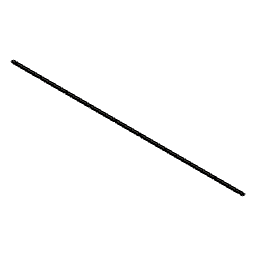
Stringers (Autodesk Fusion 360 design; units mm, degrees)
Autodesk Fusion 360 part; units mm, degrees
sketch "Sketch1" plane through (0, 0, 0) normal (0, 0, 1) x (1, 0, 0)
  line L0 (15.9527, 9.277) -> (765.9527, 9.277)
  line L1 (765.9527, 9.277) -> (765.9527, 3.277)
  line L2 (15.9527, 3.277) -> (15.9527, 9.277)
  line L3 (28.9527, 3.277) -> (28.9527, 6.277)
  line L4 (28.9527, 6.277) -> (25.9527, 6.277)
  line L5 (25.9527, 6.277) -> (25.9527, 3.277)
  line L6 (25.9527, 3.277) -> (15.9527, 3.277)
  line L7 (109.7327, 3.277) -> (109.7327, 6.277)
  line L8 (109.7327, 6.277) -> (106.7327, 6.277)
  line L9 (106.7327, 6.277) -> (106.7327, 3.277)
  line L10 (106.7327, 3.277) -> (28.9527, 3.277)
  line L11 (190.5127, 3.277) -> (190.5127, 6.277)
  line L12 (190.5127, 6.277) -> (187.5127, 6.277)
  line L13 (187.5127, 6.277) -> (187.5127, 3.277)
  line L14 (187.5127, 3.277) -> (109.7327, 3.277)
  line L15 (271.2927, 3.277) -> (271.2927, 6.277)
  line L16 (271.2927, 6.277) -> (268.2927, 6.277)
  line L17 (268.2927, 6.277) -> (268.2927, 3.277)
  line L18 (268.2927, 3.277) -> (190.5127, 3.277)
  line L19 (352.0727, 3.277) -> (352.0727, 6.277)
  line L20 (352.0727, 6.277) -> (349.0727, 6.277)
  line L21 (349.0727, 6.277) -> (349.0727, 3.277)
  line L22 (349.0727, 3.277) -> (271.2927, 3.277)
  line L23 (432.8527, 3.277) -> (432.8527, 6.277)
  line L24 (432.8527, 6.277) -> (429.8527, 6.277)
  line L25 (429.8527, 6.277) -> (429.8527, 3.277)
  line L26 (429.8527, 3.277) -> (352.0727, 3.277)
  line L27 (513.6327, 3.277) -> (513.6327, 6.277)
  line L28 (513.6327, 6.277) -> (510.6327, 6.277)
  line L29 (510.6327, 6.277) -> (510.6327, 3.277)
  line L30 (510.6327, 3.277) -> (432.8527, 3.277)
  line L31 (594.4127, 3.277) -> (594.4127, 6.277)
  line L32 (594.4127, 6.277) -> (591.4127, 6.277)
  line L33 (591.4127, 6.277) -> (591.4127, 3.277)
  line L34 (591.4127, 3.277) -> (513.6327, 3.277)
  line L35 (675.1927, 3.277) -> (675.1927, 6.277)
  line L36 (675.1927, 6.277) -> (672.1927, 6.277)
  line L37 (672.1927, 6.277) -> (672.1927, 3.277)
  line L38 (672.1927, 3.277) -> (594.4127, 3.277)
  line L39 (675.1927, 3.277) -> (752.9727, 3.277)
  line L40 (755.9727, 3.277) -> (755.9727, 6.277)
  line L41 (755.9727, 6.277) -> (752.9727, 6.277)
  line L42 (752.9727, 6.277) -> (752.9727, 3.277)
  line L43 (765.9527, 3.277) -> (755.9727, 3.277)
  line L44 (752.9727, 3.277) -> (675.1927, 3.277)
  dimension "d1" = 750
  dimension "d2" = 6
  constraint horizontal L0
  constraint vertical L1
  constraint horizontal L43
  constraint vertical L2
  constraint vertical L3
  constraint horizontal L4
  constraint vertical L5
  constraint collinear L6 L43
  constraint equal L4 L5
  constraint vertical L7
  constraint horizontal L8
  constraint vertical L9
  constraint collinear L10 L43
  constraint equal L7 L8
  constraint vertical L11
  constraint horizontal L12
  constraint vertical L13
  constraint collinear L14 L43
  constraint equal L11 L12
  constraint vertical L15
  constraint horizontal L16
  constraint vertical L17
  constraint collinear L18 L43
  constraint vertical L19
  constraint horizontal L20
  constraint vertical L21
  constraint collinear L22 L43
  constraint equal L19 L20
  constraint vertical L23
  constraint horizontal L24
  constraint vertical L25
  constraint collinear L26 L43
  constraint equal L23 L24
  constraint vertical L27
  constraint horizontal L28
  constraint vertical L29
  constraint collinear L30 L43
  constraint equal L27 L28
  constraint vertical L31
  constraint horizontal L32
  constraint vertical L33
  constraint collinear L34 L43
  constraint vertical L35
  constraint horizontal L36
  constraint vertical L37
  constraint collinear L38 L43
  constraint equal L35 L36
  constraint perpendicular L35 L39
  constraint vertical L40
  constraint horizontal L41
  constraint vertical L42
  constraint collinear L43 L44
  constraint equal L40 L41
  measures "d1" distance of L0.start L0.end
  measures "d2" distance of L0.start L2.start
extrude "Extrude1" add sketch "Sketch1" along normal blind 3
